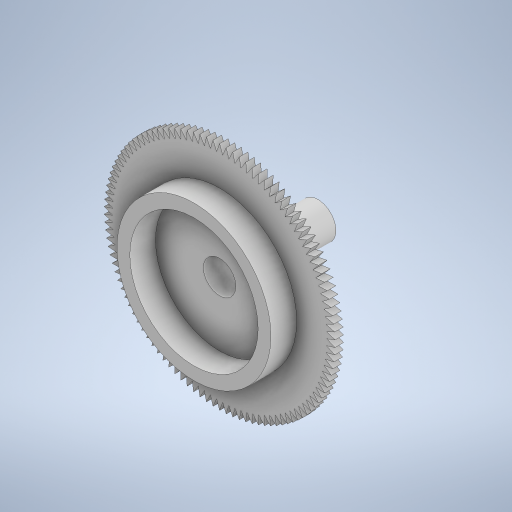
# Autodesk Inventor part: dişli
Saved by Autodesk Inventor 2023.2 (Build 272271000, 271)
## iProperties
Created: 2022-11-27
Part Number: dişli
Material: Generic
Document SubType Name: Modeling
Designer: omrfrkmll
Density: 1 g/cm^3
Appearance: Default
Author: omrfrkmll
Autodesk Inventor part; units mm, degrees
ref_plane "YZ Plane" through (0, 0, 0) normal (1, 0, 0) x (0, 1, 0)
ref_plane "XZ Plane" through (0, 0, 0) normal (0, 1, 0) x (-1, 0, 0)
ref_plane "XY Plane" through (0, 0, 0) normal (0, 0, 1) x (1, 0, 0)
sketch "Sketch2" plane through (0, 0, 0) normal (0, 0, 1) x (1, 0, 0)
  circle A0 centre (0, 0) radius 13.5
  line L0 (0, 16.2734) -> (0, -17.1435)
  line L1 (-15.0989, 0) -> (17.6929, 0)
  line L2 (0, 13.5) -> (0.364, 12.5)
  line L3 (0, 13.5) -> (-0.364, 12.5)
  line L4 (-0.7707, 13.478) -> (-1.077, 12.4588)
  line L5 (-0.7707, 13.478) -> (-0.3502, 12.5004)
  line L6 (-1.5389, 13.412) -> (-1.7865, 12.377)
  line L7 (-1.5389, 13.412) -> (-1.0633, 12.46)
  line L8 (-2.302, 13.3023) -> (-2.4902, 12.2549)
  line L9 (-2.302, 13.3023) -> (-1.7729, 12.379)
  line L10 (-3.0577, 13.1492) -> (-3.1857, 12.0927)
  line L11 (-3.0577, 13.1492) -> (-2.4767, 12.2576)
  line L12 (-3.8034, 12.9532) -> (-3.8709, 11.8911)
  line L13 (-3.8034, 12.9532) -> (-3.1724, 12.0962)
  line L14 (-4.5367, 12.7149) -> (-4.5434, 11.6507)
  line L15 (-4.5367, 12.7149) -> (-3.8578, 11.8954)
  line L16 (-5.2551, 12.4352) -> (-5.2011, 11.3724)
  line L17 (-5.2551, 12.4352) -> (-4.5306, 11.6557)
  line L18 (-5.9565, 12.1149) -> (-5.8419, 11.0569)
  line L19 (-5.9565, 12.1149) -> (-5.1886, 11.3781)
  line L20 (-6.6384, 11.7551) -> (-6.4636, 10.7053)
  line L21 (-6.6384, 11.7551) -> (-5.8297, 11.0633)
  line L22 (-7.2987, 11.3569) -> (-7.0642, 10.3189)
  line L23 (-7.2987, 11.3569) -> (-6.4518, 10.7124)
  line L24 (-7.9351, 10.9217) -> (-7.6418, 9.8988)
  line L25 (-7.9351, 10.9217) -> (-7.0529, 10.3266)
  line L26 (-8.5457, 10.4509) -> (-8.1944, 9.4464)
  line L27 (-8.5457, 10.4509) -> (-7.6309, 9.9072)
  line L28 (-9.1284, 9.946) -> (-8.7203, 8.9632)
  line L29 (-9.1284, 9.946) -> (-8.184, 9.4554)
  line L30 (-9.6813, 9.4087) -> (-9.2178, 8.4507)
  line L31 (-9.6813, 9.4087) -> (-8.7105, 8.9727)
  line L32 (-10.2026, 8.8406) -> (-9.6852, 7.9107)
  line L33 (-10.2026, 8.8406) -> (-9.2085, 8.4608)
  line L34 (-10.6907, 8.2437) -> (-10.121, 7.3449)
  line L35 (-10.6907, 8.2437) -> (-9.6765, 7.9213)
  line L36 (-11.1439, 7.62) -> (-10.5238, 6.7551)
  line L37 (-11.1439, 7.62) -> (-10.113, 7.356)
  line L38 (-11.5607, 6.9714) -> (-10.8923, 6.1433)
  line L39 (-11.5607, 6.9714) -> (-10.5164, 6.7667)
  line L40 (-11.9398, 6.3) -> (-11.2253, 5.5114)
  line L41 (-11.9398, 6.3) -> (-10.8856, 6.1552)
  line L42 (-12.28, 5.6081) -> (-11.5216, 4.8616)
  line L43 (-12.28, 5.6081) -> (-11.2192, 5.5238)
  line L44 (-12.5802, 4.8979) -> (-11.7804, 4.1959)
  line L45 (-12.5802, 4.8979) -> (-11.5162, 4.8743)
  line L46 (-12.8393, 4.1717) -> (-12.0007, 3.5166)
  line L47 (-12.8393, 4.1717) -> (-11.7757, 4.2089)
  line L48 (-13.0565, 3.4319) -> (-12.1819, 2.8257)
  line L49 (-13.0565, 3.4319) -> (-11.9968, 3.5297)
  line L50 (-13.2311, 2.681) -> (-12.3233, 2.1257)
  line L51 (-13.2311, 2.681) -> (-12.1788, 2.8391)
  line L52 (-13.3626, 1.9213) -> (-12.4246, 1.4187)
  line L53 (-13.3626, 1.9213) -> (-12.321, 2.1392)
  line L54 (-13.4505, 1.1553) -> (-12.4853, 0.7071)
  line L55 (-13.4505, 1.1553) -> (-12.423, 1.4323)
  line L56 (-13.4945, 0.3855) -> (-12.5053, -0.0069)
  line L57 (-13.4945, 0.3855) -> (-12.4845, 0.7208)
  line L58 (-13.4945, -0.3855) -> (-12.4845, -0.7208)
  line L59 (-13.4945, -0.3855) -> (-12.5053, 0.0069)
  line L60 (-13.4505, -1.1553) -> (-12.423, -1.4323)
  line L61 (-13.4505, -1.1553) -> (-12.4853, -0.7071)
  line L62 (-13.3626, -1.9213) -> (-12.321, -2.1392)
  line L63 (-13.3626, -1.9213) -> (-12.4246, -1.4187)
  line L64 (-13.2311, -2.681) -> (-12.1788, -2.8391)
  line L65 (-13.2311, -2.681) -> (-12.3233, -2.1257)
  line L66 (-13.0565, -3.4319) -> (-11.9968, -3.5297)
  line L67 (-13.0565, -3.4319) -> (-12.1819, -2.8257)
  line L68 (-12.8393, -4.1717) -> (-11.7757, -4.2089)
  line L69 (-12.8393, -4.1717) -> (-12.0007, -3.5166)
  line L70 (-12.5802, -4.8979) -> (-11.5162, -4.8743)
  line L71 (-12.5802, -4.8979) -> (-11.7804, -4.1959)
  line L72 (-12.28, -5.6081) -> (-11.2192, -5.5238)
  line L73 (-12.28, -5.6081) -> (-11.5216, -4.8616)
  line L74 (-11.9398, -6.3) -> (-10.8856, -6.1552)
  line L75 (-11.9398, -6.3) -> (-11.2253, -5.5114)
  line L76 (-11.5607, -6.9714) -> (-10.5164, -6.7667)
  line L77 (-11.5607, -6.9714) -> (-10.8923, -6.1433)
  line L78 (-11.1439, -7.62) -> (-10.113, -7.356)
  line L79 (-11.1439, -7.62) -> (-10.5238, -6.7551)
  line L80 (-10.6907, -8.2437) -> (-9.6765, -7.9213)
  line L81 (-10.6907, -8.2437) -> (-10.121, -7.3449)
  line L82 (-10.2026, -8.8406) -> (-9.2085, -8.4608)
  line L83 (-10.2026, -8.8406) -> (-9.6852, -7.9107)
  line L84 (-9.6813, -9.4087) -> (-8.7105, -8.9727)
  line L85 (-9.6813, -9.4087) -> (-9.2178, -8.4507)
  line L86 (-9.1284, -9.946) -> (-8.184, -9.4554)
  line L87 (-9.1284, -9.946) -> (-8.7203, -8.9632)
  line L88 (-8.5457, -10.4509) -> (-7.6309, -9.9072)
  line L89 (-8.5457, -10.4509) -> (-8.1944, -9.4464)
  line L90 (-7.9351, -10.9217) -> (-7.0529, -10.3266)
  line L91 (-7.9351, -10.9217) -> (-7.6418, -9.8988)
  line L92 (-7.2987, -11.3569) -> (-6.4518, -10.7124)
  line L93 (-7.2987, -11.3569) -> (-7.0642, -10.3189)
  line L94 (-6.6384, -11.7551) -> (-5.8297, -11.0633)
  line L95 (-6.6384, -11.7551) -> (-6.4636, -10.7053)
  line L96 (-5.9565, -12.1149) -> (-5.1886, -11.3781)
  line L97 (-5.9565, -12.1149) -> (-5.8419, -11.0569)
  line L98 (-5.2551, -12.4352) -> (-4.5306, -11.6557)
  line L99 (-5.2551, -12.4352) -> (-5.2011, -11.3724)
  line L100 (-4.5367, -12.7149) -> (-3.8578, -11.8954)
  line L101 (-4.5367, -12.7149) -> (-4.5434, -11.6507)
  line L102 (-3.8034, -12.9532) -> (-3.1724, -12.0962)
  line L103 (-3.8034, -12.9532) -> (-3.8709, -11.8911)
  line L104 (-3.0577, -13.1492) -> (-2.4767, -12.2576)
  line L105 (-3.0577, -13.1492) -> (-3.1857, -12.0927)
  line L106 (-2.302, -13.3023) -> (-1.7729, -12.379)
  line L107 (-2.302, -13.3023) -> (-2.4902, -12.2549)
  line L108 (-1.5389, -13.412) -> (-1.0633, -12.46)
  line L109 (-1.5389, -13.412) -> (-1.7865, -12.377)
  line L110 (-0.7707, -13.478) -> (-0.3502, -12.5004)
  line L111 (-0.7707, -13.478) -> (-1.077, -12.4588)
  line L112 (0, -13.5) -> (0.364, -12.5)
  line L113 (0, -13.5) -> (-0.364, -12.5)
  line L114 (0.7707, -13.478) -> (1.077, -12.4588)
  line L115 (0.7707, -13.478) -> (0.3502, -12.5004)
  line L116 (1.5389, -13.412) -> (1.7865, -12.377)
  line L117 (1.5389, -13.412) -> (1.0633, -12.46)
  line L118 (2.302, -13.3023) -> (2.4902, -12.2549)
  line L119 (2.302, -13.3023) -> (1.7729, -12.379)
  line L120 (3.0577, -13.1492) -> (3.1857, -12.0927)
  line L121 (3.0577, -13.1492) -> (2.4767, -12.2576)
  line L122 (3.8034, -12.9532) -> (3.8709, -11.8911)
  line L123 (3.8034, -12.9532) -> (3.1724, -12.0962)
  line L124 (4.5367, -12.7149) -> (4.5434, -11.6507)
  line L125 (4.5367, -12.7149) -> (3.8578, -11.8954)
  line L126 (5.2551, -12.4352) -> (5.2011, -11.3724)
  line L127 (5.2551, -12.4352) -> (4.5306, -11.6557)
  line L128 (5.9565, -12.1149) -> (5.8419, -11.0569)
  line L129 (5.9565, -12.1149) -> (5.1886, -11.3781)
  line L130 (6.6384, -11.7551) -> (6.4636, -10.7053)
  line L131 (6.6384, -11.7551) -> (5.8297, -11.0633)
  line L132 (7.2987, -11.3569) -> (7.0642, -10.3189)
  line L133 (7.2987, -11.3569) -> (6.4518, -10.7124)
  line L134 (7.9351, -10.9217) -> (7.6418, -9.8988)
  line L135 (7.9351, -10.9217) -> (7.0529, -10.3266)
  line L136 (8.5457, -10.4509) -> (8.1944, -9.4464)
  line L137 (8.5457, -10.4509) -> (7.6309, -9.9072)
  line L138 (9.1284, -9.946) -> (8.7203, -8.9632)
  line L139 (9.1284, -9.946) -> (8.184, -9.4554)
  line L140 (9.6813, -9.4087) -> (9.2178, -8.4507)
  line L141 (9.6813, -9.4087) -> (8.7105, -8.9727)
  line L142 (10.2026, -8.8406) -> (9.6852, -7.9107)
  line L143 (10.2026, -8.8406) -> (9.2085, -8.4608)
  line L144 (10.6907, -8.2437) -> (10.121, -7.3449)
  line L145 (10.6907, -8.2437) -> (9.6765, -7.9213)
  line L146 (11.1439, -7.62) -> (10.5238, -6.7551)
  line L147 (11.1439, -7.62) -> (10.113, -7.356)
  line L148 (11.5607, -6.9714) -> (10.8923, -6.1433)
  line L149 (11.5607, -6.9714) -> (10.5164, -6.7667)
  line L150 (11.9398, -6.3) -> (11.2253, -5.5114)
  line L151 (11.9398, -6.3) -> (10.8856, -6.1552)
  line L152 (12.28, -5.6081) -> (11.5216, -4.8616)
  line L153 (12.28, -5.6081) -> (11.2192, -5.5238)
  line L154 (12.5802, -4.8979) -> (11.7804, -4.1959)
  line L155 (12.5802, -4.8979) -> (11.5162, -4.8743)
  line L156 (12.8393, -4.1717) -> (12.0007, -3.5166)
  line L157 (12.8393, -4.1717) -> (11.7757, -4.2089)
  line L158 (13.0565, -3.4319) -> (12.1819, -2.8257)
  line L159 (13.0565, -3.4319) -> (11.9968, -3.5297)
  line L160 (13.2311, -2.681) -> (12.3233, -2.1257)
  line L161 (13.2311, -2.681) -> (12.1788, -2.8391)
  line L162 (13.3626, -1.9213) -> (12.4246, -1.4187)
  line L163 (13.3626, -1.9213) -> (12.321, -2.1392)
  line L164 (13.4505, -1.1553) -> (12.4853, -0.7071)
  line L165 (13.4505, -1.1553) -> (12.423, -1.4323)
  line L166 (13.4945, -0.3855) -> (12.5053, 0.0069)
  line L167 (13.4945, -0.3855) -> (12.4845, -0.7208)
  line L168 (13.4945, 0.3855) -> (12.4845, 0.7208)
  line L169 (13.4945, 0.3855) -> (12.5053, -0.0069)
  line L170 (13.4505, 1.1553) -> (12.423, 1.4323)
  line L171 (13.4505, 1.1553) -> (12.4853, 0.7071)
  line L172 (13.3626, 1.9213) -> (12.321, 2.1392)
  line L173 (13.3626, 1.9213) -> (12.4246, 1.4187)
  line L174 (13.2311, 2.681) -> (12.1788, 2.8391)
  line L175 (13.2311, 2.681) -> (12.3233, 2.1257)
  line L176 (13.0565, 3.4319) -> (11.9968, 3.5297)
  line L177 (13.0565, 3.4319) -> (12.1819, 2.8257)
  line L178 (12.8393, 4.1717) -> (11.7757, 4.2089)
  line L179 (12.8393, 4.1717) -> (12.0007, 3.5166)
  line L180 (12.5802, 4.8979) -> (11.5162, 4.8743)
  line L181 (12.5802, 4.8979) -> (11.7804, 4.1959)
  line L182 (12.28, 5.6081) -> (11.2192, 5.5238)
  line L183 (12.28, 5.6081) -> (11.5216, 4.8616)
  line L184 (11.9398, 6.3) -> (10.8856, 6.1552)
  line L185 (11.9398, 6.3) -> (11.2253, 5.5114)
  line L186 (11.5607, 6.9714) -> (10.5164, 6.7667)
  line L187 (11.5607, 6.9714) -> (10.8923, 6.1433)
  line L188 (11.1439, 7.62) -> (10.113, 7.356)
  line L189 (11.1439, 7.62) -> (10.5238, 6.7551)
  line L190 (10.6907, 8.2437) -> (9.6765, 7.9213)
  line L191 (10.6907, 8.2437) -> (10.121, 7.3449)
  line L192 (10.2026, 8.8406) -> (9.2085, 8.4608)
  line L193 (10.2026, 8.8406) -> (9.6852, 7.9107)
  line L194 (9.6813, 9.4087) -> (8.7105, 8.9727)
  line L195 (9.6813, 9.4087) -> (9.2178, 8.4507)
  line L196 (9.1284, 9.946) -> (8.184, 9.4554)
  line L197 (9.1284, 9.946) -> (8.7203, 8.9632)
  line L198 (8.5457, 10.4509) -> (7.6309, 9.9072)
  line L199 (8.5457, 10.4509) -> (8.1944, 9.4464)
  line L200 (7.9351, 10.9217) -> (7.0529, 10.3266)
  line L201 (7.9351, 10.9217) -> (7.6418, 9.8988)
  line L202 (7.2987, 11.3569) -> (6.4518, 10.7124)
  line L203 (7.2987, 11.3569) -> (7.0642, 10.3189)
  line L204 (6.6384, 11.7551) -> (5.8297, 11.0633)
  line L205 (6.6384, 11.7551) -> (6.4636, 10.7053)
  line L206 (5.9565, 12.1149) -> (5.1886, 11.3781)
  line L207 (5.9565, 12.1149) -> (5.8419, 11.0569)
  line L208 (5.2551, 12.4352) -> (4.5306, 11.6557)
  line L209 (5.2551, 12.4352) -> (5.2011, 11.3724)
  line L210 (4.5367, 12.7149) -> (3.8578, 11.8954)
  line L211 (4.5367, 12.7149) -> (4.5434, 11.6507)
  line L212 (3.8034, 12.9532) -> (3.1724, 12.0962)
  line L213 (3.8034, 12.9532) -> (3.8709, 11.8911)
  line L214 (3.0577, 13.1492) -> (2.4767, 12.2576)
  line L215 (3.0577, 13.1492) -> (3.1857, 12.0927)
  line L216 (2.302, 13.3023) -> (1.7729, 12.379)
  line L217 (2.302, 13.3023) -> (2.4902, 12.2549)
  line L218 (1.5389, 13.412) -> (1.0633, 12.46)
  line L219 (1.5389, 13.412) -> (1.7865, 12.377)
  line L220 (0.7707, 13.478) -> (0.3502, 12.5004)
  line L221 (0.7707, 13.478) -> (1.077, 12.4588)
  point P0 (-0.3576, -12.5175)
  point P1 (0.3576, -12.5175)
  point P2 (1.0716, -12.4767)
  point P3 (1.7822, -12.3952)
  point P4 (2.4869, -12.2732)
  point P5 (3.1835, -12.1112)
  point P6 (3.8697, -11.9097)
  point P7 (4.5433, -11.6694)
  point P8 (5.2021, -11.391)
  point P9 (5.8439, -11.0754)
  point P10 (6.4666, -10.7237)
  point P11 (7.0683, -10.3371)
  point P12 (7.6469, -9.9167)
  point P13 (8.2006, -9.464)
  point P14 (8.7275, -8.9804)
  point P15 (9.2259, -8.4675)
  point P16 (9.6943, -7.927)
  point P17 (10.131, -7.3606)
  point P18 (10.5347, -6.7702)
  point P19 (10.904, -6.1578)
  point P20 (11.2378, -5.5252)
  point P21 (11.5349, -4.8747)
  point P22 (11.7944, -4.2082)
  point P23 (12.0154, -3.528)
  point P24 (12.1972, -2.8363)
  point P25 (12.3392, -2.1354)
  point P26 (12.441, -1.4275)
  point P27 (12.5022, -0.7149)
  point P28 (12.5226, 0)
  point P29 (12.5022, 0.7149)
  point P30 (12.441, 1.4275)
  point P31 (12.3392, 2.1354)
  point P32 (12.1972, 2.8363)
  point P33 (12.0154, 3.528)
  point P34 (11.7944, 4.2082)
  point P35 (11.5349, 4.8747)
  point P36 (11.2378, 5.5252)
  point P37 (10.904, 6.1578)
  point P38 (10.5347, 6.7702)
  point P39 (10.131, 7.3606)
  point P40 (9.6943, 7.927)
  point P41 (9.2259, 8.4675)
  point P42 (8.7275, 8.9804)
  point P43 (8.2006, 9.464)
  point P44 (7.6469, 9.9167)
  point P45 (7.0683, 10.3371)
  point P46 (6.4666, 10.7237)
  point P47 (5.8439, 11.0754)
  point P48 (5.2021, 11.391)
  point P49 (4.5433, 11.6694)
  point P50 (3.8697, 11.9097)
  point P51 (3.1835, 12.1112)
  point P52 (2.4869, 12.2732)
  point P53 (1.7822, 12.3952)
  point P54 (1.0716, 12.4767)
  point P55 (0.3576, 12.5175)
  point P56 (-0.3576, 12.5175)
  point P57 (-1.0716, 12.4767)
  point P58 (-1.7822, 12.3952)
  point P59 (-2.4869, 12.2732)
  point P60 (-3.1835, 12.1112)
  point P61 (-3.8697, 11.9097)
  point P62 (-4.5433, 11.6694)
  point P63 (-5.2021, 11.391)
  point P64 (-5.8439, 11.0754)
  point P65 (-6.4666, 10.7237)
  point P66 (-7.0683, 10.3371)
  point P67 (-7.6469, 9.9167)
  point P68 (-8.2006, 9.464)
  point P69 (-8.7275, 8.9804)
  point P70 (-9.2259, 8.4675)
  point P71 (-9.6943, 7.927)
  point P72 (-10.131, 7.3606)
  point P73 (-10.5347, 6.7702)
  point P74 (-10.904, 6.1578)
  point P75 (-11.2378, 5.5252)
  point P76 (-11.5349, 4.8747)
  point P77 (-11.7944, 4.2082)
  point P78 (-12.0154, 3.528)
  point P79 (-12.1972, 2.8363)
  point P80 (-12.3392, 2.1354)
  point P81 (-12.441, 1.4275)
  point P82 (-12.5022, 0.7149)
  point P83 (-12.5226, 0)
  point P84 (-12.5022, -0.7149)
  point P85 (-12.441, -1.4275)
  point P86 (-12.3392, -2.1354)
  point P87 (-12.1972, -2.8363)
  point P88 (-12.0154, -3.528)
  point P89 (-11.7944, -4.2082)
  point P90 (-11.5349, -4.8747)
  point P91 (-11.2378, -5.5252)
  point P92 (-10.904, -6.1578)
  point P93 (-10.5347, -6.7702)
  point P94 (-10.131, -7.3606)
  point P95 (-9.6943, -7.927)
  point P96 (-9.2259, -8.4675)
  point P97 (-8.7275, -8.9804)
  point P98 (-8.2006, -9.464)
  point P99 (-7.6469, -9.9167)
  point P100 (-7.0683, -10.3371)
  point P101 (-6.4666, -10.7237)
  point P102 (-5.8439, -11.0754)
  point P103 (-5.2021, -11.391)
  point P104 (-4.5433, -11.6694)
  point P105 (-3.8697, -11.9097)
  point P106 (-3.1835, -12.1112)
  point P107 (-2.4869, -12.2732)
  point P108 (-1.7822, -12.3952)
  point P109 (-1.0716, -12.4767)
  dimension "d7" = 27
  dimension "d8" = 40
  dimension "d9" = 12.5
  dimension "d12" = 360
  constraints: 444 end point, 2 horizontal, 2 vertical, 1 coincident, 1 point on line, 1 symmetric about line, 1 vertical alignment, 554 other
  measures "d8" angle of L2 L3
  measures "d9" vertical distance of point (0, 0) L2.end
extrude "Extrusion1" add sketch "Sketch2" against normal blind 1 contours L169 L1 L0 L2 L220 L221 L218 L219 L216 L217 L214 L215 L212 L213 L210 L211 L208 L209 L206 L207 L204 L205 L202 L203 L200 L201 L198 L199 L196 L197 L194 L195 L192 L193 L190 L191 L188 L189 L186 L187 L184 L185 L182 L183 L180 L181 L178 L179 L176 L177 L174 L175 L172 L173 L170 L171 L168 | L167 L164 L165 L162 L163 L160 L161 L158 L159 L156 L157 L154 L155 L152 L153 L150 L151 L148 L149 L146 L147 L144 L145 L142 L143 L140 L141 L138 L139 L136 L137 L134 L135 L132 L133 L130 L131 L128 L129 L126 L127 L124 L125 L122 L123 L120 L121 L118 L119 L116 L117 L114 L115 L112 L0 L1 L166 | L1 L56 L57 L54 L55 L52 L53 L50 L51 L48 L49 L46 L47 L44 L45 L42 L43 L40 L41 L38 L39 L36 L37 L34 L35 L32 L33 L30 L31 L28 L29 L26 L27 L24 L25 L22 L23 L20 L21 L18 L19 L16 L17 L14 L15 L12 L13 L10 L11 L8 L9 L6 L7 L4 L5 L3 L0 | L0 L113 L110 L111 L108 L109 L106 L107 L104 L105 L102 L103 L100 L101 L98 L99 L96 L97 L94 L95 L92 L93 L90 L91 L88 L89 L86 L87 L84 L85 L82 L83 L80 L81 L78 L79 L76 L77 L74 L75 L72 L73 L70 L71 L68 L69 L66 L67 L64 L65 L62 L63 L60 L61 L58 L59 L1
sketch "Sketch3" plane through (0, 0, 0) normal (0, 0, 1) x (1, 0, 0)
  circle A0 centre (0, 0) radius 1.9
  dimension "d16" = 3.8
  constraints: 1 centre point, 1 coincident
  measures "d16" diameter of A0
extrude "Extrusion2" cut sketch "Sketch3" against normal through all
sketch "Sketch4" plane through (0, 0, 0) normal (0, 0, 1) x (1, 0, 0)
  circle A0 centre (0, 0) radius 9
  circle A1 centre (0, 0) radius 7.5
  dimension "d19" = 18
  dimension "d22" = 1.5
  constraints: 2 centre point, 1 coincident
  measures "d19" diameter of A0
  measures "d22" radial gap between concentric circles of A0 A1
extrude "Extrusion3" add sketch "Sketch4" along normal blind 3
sketch "Sketch6" plane through (0, 0, -1) normal (0, 0, -1) x (-1, 0, 0)
  circle A0 centre (0, 0) radius 1.9
  circle A1 centre (0, 0) radius 1.9 projected
  circle A2 centre (0, 0) radius 4.5
  dimension "d23" = 9
  constraints: 2 centre point, 2 coincident
  measures "d23" diameter of A2
extrude "Extrusion4" add sketch "Sketch6" along normal blind 4.5
fillet "Fillet1" radius 2 1 edges at (4.5, 0, -1)
sketch "Sketch7" plane through (0, 0, -5.5) normal (0, 0, -1) x (-1, 0, 0)
  circle A0 centre (0, 0) radius 1.9 projected
  circle A1 centre (0, 0) radius 1.9
  circle A2 centre (0, 0) radius 2.1
  dimension "d27" = 0.2
  constraints: 2 centre point, 1 coincident
  measures "d27" radial gap between concentric circles of A0 A2
extrude "Extrusion5" add sketch "Sketch7" along normal blind 6
body "Solid1"
